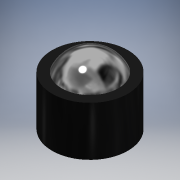
# Autodesk Inventor part: Caster
Saved by Autodesk Inventor 2019 (Build 230136000, 136)
## iProperties
Created: 2019-01-28
Part Number: Caster
Material: Generic
Document SubType Name: Modeling
Designer: scigu
Density: 1 g/cm^3
Appearance: Default
Mass: 6.9115 g
Surface Area: 20.8837 cm^2
Volume: 6.9115 cm^3
Author: scigu
Autodesk Inventor part; units mm, degrees
ref_plane "YZ Plane" through (0, 0, 0) normal (1, 0, 0) x (0, 1, 0)
ref_plane "XZ Plane" through (0, 0, 0) normal (0, 1, 0) x (-1, 0, 0)
ref_plane "XY Plane" through (0, 0, 0) normal (0, 0, 1) x (1, 0, 0)
sketch "Sketch1" plane through (0, 0, 0) normal (0, 1, 0) x (-1, 0, 0)
  circle A0 centre (0, 0) radius 11.5
  dimension "d0" = 23
  constraints: 1 centre point, 1 coincident
  measures "d0" diameter of A0
extrude "Extrusion1" add sketch "Sketch1" along normal blind 15
sketch "Sketch2" plane through (0, 0, 0) normal (1, 0, 0) x (0, 1, 0)
  line L0 (0, 0) -> (20.5, 0)
  line L1 (20.5, 0) -> (11.0014, 0) construction
  line L2 (20.5, 0) -> (29.9986, 0) construction
  arc A0 (20.5, 0) -> (15, 8.616) centre (11.0014, 0) ccw
  line L3 (15, 8.616) -> (15, 0)
  line L4 (15, -11.5) -> (15, 11.5) projected
  line L5 (15, 8.616) -> (15, 0)
  line L6 (20.5, 0) -> (15, 0)
  arc A1 (20.5, 0) -> (15, 8.616) centre (11.0014, 0) ccw
  dimension "d3" = 20.5
  dimension "d4" = 9.4986
  dimension "d5" = 180
  constraints: 12 end point, 4 point on circle, 2 centre point, 2 coincident, 2 collinear, 2 horizontal, 1 midpoint, 1 perpendicular, 1 vertical
  measures "d3" distance of L0.start L0.end
  measures "d4" distance of L0.end L1.end
  measures "d5" angle of L1 L2
revolve "Revolution1" add sketch "Sketch2" angle 360 about axis through (0, 20.5, 0) along (0, 1, 0)
sketch "Sketch3" plane through (0, 0, 0) normal (0, -1, 0) x (1, 0, 0)
  line L0 (0, 0) -> (0, -7.5) construction
  line L1 (0, -7.5) -> (0, 7.5)
  circle A0 centre (0, 7.5) radius 1.25
  circle A1 centre (0, -7.5) radius 1.25
  dimension "d7" = 7.5
  dimension "d8" = 15
  dimension "d9" = 2.5
  dimension "d10" = 2.5
  constraints: 4 end point, 2 centre point, 2 coincident, 1 point on line, 1 vertical
  measures "d7" distance of L0.start L0.end
  measures "d8" distance of L0.end L1.end
  measures "d9" diameter of A0
  measures "d10" diameter of A1
extrude "Extrusion2" cut sketch "Sketch3" against normal blind 5
body "Solid1"
